Autodesk Fusion 360 part; units mm, degrees
(part 3 of 4)
extrude "Extrude14" cut sketch "left_side_misc" along normal up to surface (5.36 mm away) from surface at 107.32 contours A0 | A1 | A2 bodies 9
sketch "layer_0" plane through (0, 0, 0) normal (0, 1, 0) x (1, 0, 0)
  line L0 (-84.68, -41.5) -> (77.32, -41.5)
  line L1 (77.32, -41.5) -> (77.32, 105.5) construction
  line L2 (77.32, 105.5) -> (-84.68, 105.5)
  line L3 (-84.68, 105.5) -> (-84.68, -41.5)
  line L4 (38.25, 90) -> (38.25, -6)
  line L5 (38.25, 90) -> (77.32, 90)
  line L6 (38.25, -6) -> (77.32, -6)
  line L7 (77.32, 90) -> (77.32, 105.5)
  line L8 (77.32, -6) -> (77.32, -41.5)
  line L9 (72.32, -41.5) -> (72.32, -21.5) construction
  line L10 (72.32, -21.5) -> (77.32, -21.5) construction
  line L11 (-79.68, -41.5) -> (-79.68, -21.5) construction
  line L12 (-79.68, -21.5) -> (-84.68, -21.5) construction
  line L13 (-100, 100) -> (100, 100) construction
  line L14 (77.32, -6) -> (70.32, -6) construction
  line L15 (70.32, -6) -> (70.32, -13) construction
  line L16 (70.32, -13) -> (77.32, -13) construction
  line L17 (77.32, -13) -> (77.32, -6) construction
  line L18 (77.32, 90) -> (70.32, 90) construction
  line L19 (70.32, 90) -> (70.32, 97) construction
  line L20 (70.32, 97) -> (77.32, 97) construction
  line L21 (77.32, 97) -> (77.32, 90) construction
  line L22 (38.25, 90) -> (31.25, 90) construction
  line L23 (31.25, 90) -> (31.25, 97) construction
  line L24 (31.25, 97) -> (38.25, 97) construction
  line L25 (38.25, 97) -> (38.25, 90) construction
  line L26 (38.25, -6) -> (31.25, -6) construction
  line L27 (31.25, -6) -> (31.25, -13) construction
  line L28 (31.25, -13) -> (38.25, -13) construction
  line L29 (38.25, -13) -> (38.25, -6) construction
  line L30 (38.25, 97) -> (70.32, 97) construction
  line L31 (31.25, 90) -> (31.25, -6) construction
  line L32 (38.25, -13) -> (70.32, -13) construction
  line L33 (77.32, -9.5) -> (34.75, -9.5) construction
  line L34 (77.32, 93.5) -> (34.75, 93.5) construction
  line L35 (34.75, 93.5) -> (34.75, -9.5) construction
  line L36 (73.82, -9.5) -> (73.82, -13) construction
  line L37 (73.82, 97) -> (73.82, 93.5) construction
  line L38 (31.25, 97) -> (21.32, 97) construction
  line L39 (21.32, 97) -> (21.32, -13) construction
  line L40 (21.32, -13) -> (31.25, -13) construction
  line L41 (21.32, 42) -> (28.32, 42) construction
  line L42 (21.32, 5) -> (77.32, 5) construction
  line L43 (77.32, 90) -> (73.82, 90) construction
  line L44 (73.82, 90) -> (73.82, 86.5) construction
  line L45 (73.82, 86.5) -> (77.32, 86.5) construction
  line L46 (77.32, 86.5) -> (77.32, 90) construction
  line L47 (73.82, 86.5) -> (24.82, 86.5) construction
  line L48 (24.82, 86.5) -> (24.82, 28.5) construction
  line L49 (24.82, 28.5) -> (73.82, 28.5) construction
  line L50 (73.82, 28.5) -> (73.82, 86.5) construction
  line L51 (-84.68, 90) -> (-36.68, 90) construction
  line L52 (-36.68, 90) -> (-36.68, 21) construction
  line L53 (-36.68, 21) -> (-84.68, 21) construction
  line L54 (-84.68, 21) -> (-84.68, 90) construction
  line L55 (31.25, 90) -> (-84.68, 90) construction
  line L56 (-39.62, 23.94) -> (-81.74, 23.94) construction
  line L57 (-81.74, 23.94) -> (-81.74, 87.06) construction
  line L58 (-81.74, 87.06) -> (-39.62, 87.06) construction
  line L59 (-39.62, 87.06) -> (-39.62, 23.94) construction
  line L60 (-84.68, 90) -> (-81.74, 90) construction
  line L61 (-81.74, 90) -> (-81.74, 87.06) construction
  line L62 (-81.74, 87.06) -> (-84.68, 87.06) construction
  line L63 (-84.68, 87.06) -> (-84.68, 90) construction
  line L64 (-39.62, 23.94) -> (-36.68, 23.94) construction
  line L65 (-36.68, 23.94) -> (-36.68, 21) construction
  line L66 (-36.68, 21) -> (-39.62, 21) construction
  line L67 (-39.62, 21) -> (-39.62, 23.94) construction
  line L68 (-33.68, 17.618) -> (-1.422, 17.618) construction
  line L69 (-1.422, 17.618) -> (-1.422, -37.5) construction
  line L70 (-1.422, -37.5) -> (-33.68, -37.5) construction
  line L71 (-33.68, -37.5) -> (-33.68, 17.618) construction
  line L72 (-4.851, -34.071) -> (-30.251, -34.071) construction
  line L73 (-30.251, -34.071) -> (-30.251, 14.189) construction
  line L74 (-30.251, 14.189) -> (-4.851, 14.189) construction
  line L75 (-4.851, 14.189) -> (-4.851, -34.071) construction
  point P0 (-84.68, -41.5)
  point P1 (77.32, 105.5)
  point P2 (34.75, -6)
  point P3 (73.82, -9.5)
  point P4 (73.82, 93.5)
  point P5 (24.82, 42)
  dimension "d299" = 7
  dimension "d300" = 56
  dimension "d301" = 7
  dimension "d303" = 85
  dimension "d304" = 3.5
  dimension "d305" = 3.5
  dimension "d306" = 49
  dimension "d307" = 58
  dimension "d326" = 48
  dimension "d327" = 69
  dimension "d328" = 2.94
  dimension "d404" = 32.258
  dimension "d405" = 55.118
  dimension "d406" = 3.429
  dimension "d407" = 4
  dimension "d408" = 3
  constraint horizontal L0
  constraint vertical L1
  constraint horizontal L2
  constraint vertical L3
  constraint coincident P1 L1.end
  constraint coincident P0 L0.start
  constraint coincident L4.start L5.start
  constraint coincident L1 L5.end
  constraint perpendicular L1 L5
  constraint coincident L4.end L6.start
  constraint coincident L1 L6.end
  constraint perpendicular L1 L6
  constraint horizontal L14
  constraint vertical L15
  constraint horizontal L16
  constraint vertical L17
  constraint equal L15 L16
  constraint horizontal L18
  constraint vertical L19
  constraint horizontal L20
  constraint vertical L21
  constraint equal L19 L20
  constraint equal L15 L19
  constraint horizontal L22
  constraint vertical L23
  constraint horizontal L24
  constraint vertical L25
  constraint horizontal L26
  constraint vertical L27
  constraint horizontal L28
  constraint vertical L29
  constraint equal L15 L29
  constraint equal L26 L29
  constraint equal L22 L26
  constraint equal L22 L25
  constraint midpoint L17 L33.start
  constraint perpendicular L17 L33
  constraint midpoint L21 L34.start
  constraint perpendicular L25 L34
  constraint vertical L35
  constraint midpoint L26 P2
  constraint coincident L35 P2
  constraint coincident L33 P3
  constraint coincident P3 L36.start
  constraint midpoint L16 L36.end
  constraint vertical L36
  constraint midpoint L20 L37.start
  constraint coincident L34 P4
  constraint perpendicular L34 L37
  constraint coincident P4 L37.end
  constraint perpendicular L23 L38
  constraint perpendicular L22 L39
  constraint horizontal L40
  constraint midpoint L39 L41.start
  constraint perpendicular L39 L41
  constraint midpoint L41 P5
  constraint coincident L39 L42.start
  constraint coincident L1 L42.end
  constraint perpendicular L1 L42
  constraint horizontal L43
  constraint vertical L44
  constraint horizontal L45
  constraint vertical L46
  constraint horizontal L47
  constraint vertical L48
  constraint horizontal L49
  constraint vertical L50
  constraint coincident L3 L51.start
  constraint horizontal L51
  constraint vertical L52
  constraint horizontal L53
  constraint vertical L54
  constraint perpendicular L3 L55
  constraint coincident L51.start L54.end
  constraint horizontal L56
  constraint vertical L57
  constraint horizontal L58
  constraint vertical L59
  constraint horizontal L60
  constraint vertical L61
  constraint horizontal L62
  constraint vertical L63
  constraint horizontal L64
  constraint vertical L65
  constraint horizontal L66
  constraint vertical L67
  constraint equal L64 L67
  constraint equal L62 L64
  constraint equal L61 L62
  constraint horizontal L68
  constraint vertical L69
  constraint horizontal L70
  constraint vertical L71
  measures "d299" distance of L6.end L16.end
  measures "d300" distance of L20.end L38.end
  measures "d301" distance of L41.start L41.end
  measures "d303" distance of L5 L42
  measures "d304" distance of L5.end L43.end
  measures "d305" distance of L5.end L45.end
  measures "d306" distance of L44.end L47.end
  measures "d307" distance of L44.end L49.end
  measures "d326" distance of L51.start L51.end
  measures "d327" distance of L51.start L53.end
  measures "d328" distance of L56.start L66.end
  measures "d404" distance of L68.start L68.end
  measures "d405" distance of L68.end L69.end
  measures "d407" distance of L0 L70
  measures "d408" distance of L52 L71
sketch "layer_0_rpi_adapter" plane through (0, 0, 0) normal (0, 1, 0) x (1, 0, 0)
  line L0 (21.32, 97) -> (77.32, 97)
  line L1 (77.32, 97) -> (77.32, -13)
  line L2 (77.32, -13) -> (21.32, -13)
  line L3 (21.32, -13) -> (21.32, 97)
  line L4 (21.32, -13) -> (3.32, -13) construction
  line L5 (3.32, -13) -> (3.32, 97) construction
  line L6 (3.32, 97) -> (21.32, 97) construction
  point P0 (21.32, 97)
  point P1 (77.32, -13)
  dimension "d325" = 18
  constraint horizontal L0
  constraint vertical L1
  constraint horizontal L2
  constraint vertical L3
  constraint coincident P1 L1.end
  constraint coincident P0 L0.start
  constraint perpendicular L3 L4
  constraint perpendicular L4 L5
  constraint horizontal L6
  measures "d325" distance of L2.end L4.end
sketch "layer 0 planning" plane through (0, 0, 0) normal (0, 0, 1) x (1, 0, 0)
  line L0 (100, 42.675) -> (-100, 42.675)
  line L1 (100, 37.325) -> (-100, 37.325)
  line L2 (77.32, 42.675) -> (21.32, 42.675)
  line L3 (21.32, 42.675) -> (21.32, 47.675)
  line L4 (21.32, 47.675) -> (77.32, 47.675)
  line L5 (77.32, 47.675) -> (77.32, 42.675)
  line L6 (77.32, 47.675) -> (21.32, 47.675)
  line L7 (21.32, 47.675) -> (21.32, 53.025)
  line L8 (21.32, 53.025) -> (77.32, 53.025)
  line L9 (77.32, 53.025) -> (77.32, 47.675)
  line L10 (77.32, 53.025) -> (21.32, 53.025)
  line L11 (21.32, 53.025) -> (21.32, 58.025)
  line L12 (21.32, 58.025) -> (77.32, 58.025)
  line L13 (77.32, 58.025) -> (77.32, 53.025)
  line L14 (77.32, 58.025) -> (21.32, 58.025)
  line L15 (21.32, 58.025) -> (21.32, 76.025)
  line L16 (21.32, 76.025) -> (77.32, 76.025)
  line L17 (77.32, 76.025) -> (77.32, 58.025)
  point P0 (77.32, 0)
  point P1 (21.32, 0)
  dimension "d315" = 5
  dimension "d316" = 5.35
  dimension "d317" = 5
  dimension "d318" = 18
  constraint horizontal L2
  constraint vertical L3
  constraint horizontal L4
  constraint vertical L5
  constraint coincident L0 L2.start
  constraint vertical P1 L2.end
  constraint vertical P0 L2.start
  constraint horizontal L6
  constraint vertical L7
  constraint horizontal L8
  constraint vertical L9
  constraint vertical L3.end L7.end
  constraint horizontal L10
  constraint vertical L11
  constraint horizontal L12
  constraint vertical L13
  constraint vertical L7.end L11.end
  constraint horizontal L14
  constraint vertical L15
  constraint horizontal L16
  constraint vertical L17
  constraint vertical L11.end L15.end
  measures "d315" distance of L2.start L4.end
  measures "d316" distance of L4.end L8.end
  measures "d317" distance of L8.end L12.end
  measures "d318" distance of L12.end L16.end
extrude "Extrude21" add sketch "layer_0_rpi_adapter" along normal up to surface (5.35 mm away) from surface at 47.675 separate body makes body 12
extrude "Extrude22" add sketch "layer_0" along normal up to surface (5.35 mm away) from surface at 37.325 separate body makes body 13
hole "Hole6" at (73.82, 0, 9.5) at (34.75, 0, 9.5) at (24.82, 0, -42) at (34.75, 0, -93.5) at (73.82, 0, -93.5) at (-39.62, 0, -23.94) at (-39.62, 0, -87.06) at (-81.74, 0, -23.94) at (-81.74, 0, -87.06) at (-4.851, 0, 34.071) at (-4.851, 0, -14.189) at (-30.251, 0, -14.189) at (-30.251, 0, 34.071) direction (0, 1, 0) diameter 1.8 end up to surface (42.675 mm away) bodies 13
hole "Hole7" at (34.75, 0, -93.5) at (73.82, 0, -93.5) at (34.75, 0, 9.5) at (73.82, 0, 9.5) at (24.82, 0, -42) direction (0, 1, 0) diameter 2.8 end up to surface (53.025 mm away) bodies 4 12
hole "Hole8" at (24.82, 0, -86.5) at (24.82, 0, -28.5) at (73.82, 0, -28.5) at (73.82, 0, -86.5) direction (0, 1, 0) diameter 1.8 end up to surface (53.025 mm away) bodies 12
sketch "layer_0_laser" plane through (0, 42.675, 0) normal (0, 1, 0) x (-1, 0, 0)
  circle A0 centre (81.74, -23.94) radius 0.9
  circle A1 centre (39.62, -23.94) radius 0.9
  circle A2 centre (-34.75, -93.5) radius 0.9
  circle A3 centre (-34.75, 9.5) radius 0.9
  circle A4 centre (-73.82, 9.5) radius 0.9
  circle A5 centre (-24.82, -42) radius 0.9
  circle A6 centre (-73.82, -93.5) radius 0.9
  circle A7 centre (39.62, -87.06) radius 0.9
  circle A8 centre (81.74, -87.06) radius 0.9
  line L0 (-38.25, 6) -> (-38.25, -90)
  line L1 (-38.25, -90) -> (-77.32, -90)
  line L2 (-77.32, -90) -> (-77.32, -105.5)
  line L3 (-77.32, -105.5) -> (84.68, -105.5)
  line L4 (84.68, -105.5) -> (84.68, 41.5)
  line L5 (84.68, 41.5) -> (-77.32, 41.5)
  line L6 (-77.32, 41.5) -> (-77.32, 6)
  line L7 (-77.32, 6) -> (-38.25, 6)
  circle A9 centre (30.251, -14.189) radius 0.9
  circle A10 centre (4.851, 34.071) radius 0.9
  circle A11 centre (4.851, -14.189) radius 0.9
  circle A12 centre (30.251, 34.071) radius 0.9
sketch "layer_0_rpi_adapter_laser" plane through (0, 53.025, 0) normal (0, 1, 0) x (-1, 0, 0)
  circle A0 centre (-73.82, -28.5) radius 0.9
  circle A1 centre (-24.82, -86.5) radius 0.9
  circle A2 centre (-24.82, -28.5) radius 0.9
  circle A3 centre (-73.82, -86.5) radius 0.9
  circle A4 centre (-73.82, 9.5) radius 1.4
  circle A5 centre (-73.82, -93.5) radius 1.4
  circle A6 centre (-34.75, -93.5) radius 1.4
  circle A7 centre (-34.75, 9.5) radius 1.4
  circle A8 centre (-24.82, -42) radius 1.4
  line L0 (-21.32, -97) -> (-21.32, 13)
  line L1 (-21.32, 13) -> (-77.32, 13)
  line L2 (-77.32, 13) -> (-77.32, -97)
  line L3 (-77.32, -97) -> (-21.32, -97)
sketch "right_panel_laser" plane through (-112.68, 0, 0) normal (-1, 0, 0) x (0, 0, 1)
  circle A0 centre (32.8, 120) radius 2.5
  circle A1 centre (32.8, 199.925) radius 2.5
  circle A2 centre (32.8, 40.075) radius 2.5
  circle A3 centre (61, 170.495) radius 5
  circle A4 centre (37, 170.495) radius 5
  circle A5 centre (67, 180.8873) radius 5
  circle A6 centre (85, 191.28) radius 5
  circle A7 centre (85, 170.495) radius 5
  circle A8 centre (67, 139.3173) radius 5
  circle A9 centre (67, 118.5323) radius 5
  circle A10 centre (67, 97.7473) radius 5
  circle A11 centre (61, 108.14) radius 5
  circle A12 centre (55, 139.3173) radius 5
  circle A13 centre (49, 149.71) radius 5
  circle A14 centre (31, 160.1023) radius 5
  circle A15 centre (55, 160.1023) radius 5
  circle A16 centre (79, 160.1023) radius 5
  circle A17 centre (79, 139.3173) radius 5
  circle A18 centre (79, 118.5323) radius 5
  circle A19 centre (79, 97.7473) radius 5
  circle A20 centre (85, 87.355) radius 5
  circle A21 centre (85, 66.57) radius 5
  circle A22 centre (61, 87.355) radius 5
  circle A23 centre (67, 76.9623) radius 5
  circle A24 centre (61, 66.57) radius 5
  circle A25 centre (49, 66.57) radius 5
  circle A26 centre (67, 56.1773) radius 5
  circle A27 centre (85, 45.785) radius 5
  circle A28 centre (85, 25) radius 5
  circle A29 centre (61, 45.785) radius 5
  circle A30 centre (61, 25) radius 5
  circle A31 centre (37, 25) radius 5
  circle A32 centre (55, 35.3923) radius 5
  circle A33 centre (43, 56.1773) radius 5
  circle A34 centre (25, 66.57) radius 5
  circle A35 centre (49, 87.355) radius 5
  circle A36 centre (31, 76.9623) radius 5
  circle A37 centre (37, 87.355) radius 5
  circle A38 centre (19, 97.7473) radius 5
  circle A39 centre (43, 97.7473) radius 5
  circle A40 centre (55, 118.5323) radius 5
  circle A41 centre (43, 139.3173) radius 5
  circle A42 centre (19, 139.3173) radius 5
  circle A43 centre (19, 160.1023) radius 5
  circle A44 centre (19, 180.8873) radius 5
  circle A45 centre (43, 180.8873) radius 5
  circle A46 centre (61, 191.28) radius 5
  circle A47 centre (49, 191.28) radius 5
  circle A48 centre (31, 180.8873) radius 5
  circle A49 centre (25, 170.495) radius 5
  circle A50 centre (25, 149.71) radius 5
  circle A51 centre (31, 139.3173) radius 5
  circle A52 centre (49, 128.925) radius 5
  circle A53 centre (49, 108.14) radius 5
  circle A54 centre (31, 97.7473) radius 5
  circle A55 centre (25, 87.355) radius 5
  circle A56 centre (19, 76.9623) radius 5
  circle A57 centre (43, 76.9623) radius 5
  circle A58 centre (19, 56.1773) radius 5
  circle A59 centre (31, 56.1773) radius 5
  circle A60 centre (49, 45.785) radius 5
  circle A61 centre (49, 25) radius 5
  circle A62 centre (25, 25) radius 5
  circle A63 centre (67, 35.3923) radius 5
  circle A64 centre (73, 25) radius 5
  circle A65 centre (79, 35.3923) radius 5
  circle A66 centre (73, 45.785) radius 5
  circle A67 centre (55, 56.1773) radius 5
  circle A68 centre (37, 66.57) radius 5
  circle A69 centre (55, 76.9623) radius 5
  circle A70 centre (73, 66.57) radius 5
  circle A71 centre (79, 56.1773) radius 5
  circle A72 centre (79, 76.9623) radius 5
  circle A73 centre (73, 87.355) radius 5
  circle A74 centre (85, 108.14) radius 5
  circle A75 centre (85, 128.925) radius 5
  circle A76 centre (85, 149.71) radius 5
  circle A77 centre (67, 160.1023) radius 5
  circle A78 centre (43, 160.1023) radius 5
  circle A79 centre (37, 149.71) radius 5
  circle A80 centre (61, 149.71) radius 5
  circle A81 centre (61, 128.925) radius 5
  circle A82 centre (55, 97.7473) radius 5
  circle A83 centre (73, 108.14) radius 5
  circle A84 centre (73, 128.925) radius 5
  circle A85 centre (73, 149.71) radius 5
  circle A86 centre (79, 180.8873) radius 5
  circle A87 centre (73, 191.28) radius 5
  circle A88 centre (55, 180.8873) radius 5
  circle A89 centre (49, 170.495) radius 5
  circle A90 centre (73, 170.495) radius 5
  line L0 (105.5, 215.5) -> (-105.5, 215.5)
  line L1 (-105.5, 215.5) -> (-105.5, 4.5)
  line L2 (-105.5, 4.5) -> (105.5, 4.5)
  line L3 (105.5, 4.5) -> (105.5, 215.5)
sketch "left_panel_laser" plane through (112.68, 0, 0) normal (1, 0, 0) x (0, 0, -1)
  circle A0 centre (-64, 29.5) radius 11.6
  circle A1 centre (-73.6, 41.5) radius 1.1
  circle A2 centre (-54.4, 17.5) radius 1.1
  circle A3 centre (-34.3, 120) radius 2.5
  circle A4 centre (-34.3, 199.925) radius 2.5
  circle A5 centre (-34.3, 40.075) radius 2.5
  line L0 (-105.5, 215.5) -> (-105.5, 4.5)
  line L1 (-105.5, 4.5) -> (105.5, 4.5)
  line L2 (105.5, 4.5) -> (105.5, 215.5)
  line L3 (105.5, 215.5) -> (-105.5, 215.5)
  circle A6 centre (14.25, 188.25) radius 2.5
  line L4 (10, 135.4047) -> (10, 169.5953)
  arc A7 (32.9047, 192.5) -> (10, 169.5953) centre (50, 152.5) ccw
  line L5 (32.9047, 192.5) -> (67.0953, 192.5)
  arc A8 (90, 169.5953) -> (67.0953, 192.5) centre (50, 152.5) ccw
  line L6 (90, 169.5953) -> (90, 135.4047)
  arc A9 (67.0953, 112.5) -> (90, 135.4047) centre (50, 152.5) ccw
  line L7 (67.0953, 112.5) -> (32.9047, 112.5)
  arc A10 (10, 135.4047) -> (32.9047, 112.5) centre (50, 152.5) ccw
  circle A11 centre (85.75, 90.75) radius 2.5
  circle A12 centre (85.75, 188.25) radius 2.5
  circle A13 centre (14.25, 90.75) radius 2.5
  circle A14 centre (14.25, 116.75) radius 2.5
  circle A15 centre (85.75, 116.75) radius 2.5
  arc A16 (32.9047, 95) -> (10, 72.0953) centre (50, 55) ccw
  line L8 (32.9047, 95) -> (67.0953, 95)
  arc A17 (90, 72.0953) -> (67.0953, 95) centre (50, 55) ccw
  line L9 (90, 72.0953) -> (90, 37.9047)
  arc A18 (67.0953, 15) -> (90, 37.9047) centre (50, 55) ccw
  line L10 (67.0953, 15) -> (32.9047, 15)
  arc A19 (10, 37.9047) -> (32.9047, 15) centre (50, 55) ccw
  line L11 (10, 37.9047) -> (10, 72.0953)
  circle A20 centre (14.25, 19.25) radius 2.5
  circle A21 centre (85.75, 19.25) radius 2.5
sketch "left_panel_pcb_plan" plane through (107.32, 0, 0) normal (-1, 0, 0) x (0, 0, 1)
  circle A0 centre (64, 29.5) radius 11.6
  circle A1 centre (73.6, 41.5) radius 1.1
  circle A2 centre (54.4, 17.5) radius 1.1
  circle A3 centre (34.3, 120) radius 2.5
  circle A4 centre (34.3, 199.925) radius 2.5
  circle A5 centre (34.3, 40.075) radius 2.5
  circle A6 centre (-14.25, 188.25) radius 2.5
  arc A7 (-10, 169.5953) -> (-32.9047, 192.5) centre (-50, 152.5) ccw
  line L0 (-10, 169.5953) -> (-10, 135.4047)
  arc A8 (-32.9047, 112.5) -> (-10, 135.4047) centre (-50, 152.5) ccw
  line L1 (-32.9047, 112.5) -> (-67.0953, 112.5)
  arc A9 (-90, 135.4047) -> (-67.0953, 112.5) centre (-50, 152.5) ccw
  line L2 (-90, 135.4047) -> (-90, 169.5953)
  arc A10 (-67.0953, 192.5) -> (-90, 169.5953) centre (-50, 152.5) ccw
  line L3 (-67.0953, 192.5) -> (-32.9047, 192.5)
  circle A11 centre (-85.75, 90.75) radius 2.5
  circle A12 centre (-85.75, 188.25) radius 2.5
  circle A13 centre (-14.25, 90.75) radius 2.5
  circle A14 centre (-14.25, 116.75) radius 2.5
  circle A15 centre (-85.75, 116.75) radius 2.5
  line L4 (-67.0953, 95) -> (-32.9047, 95)
  arc A16 (-10, 72.0953) -> (-32.9047, 95) centre (-50, 55) ccw
  line L5 (-10, 72.0953) -> (-10, 37.9047)
  arc A17 (-32.9047, 15) -> (-10, 37.9047) centre (-50, 55) ccw
  line L6 (-32.9047, 15) -> (-67.0953, 15)
  arc A18 (-90, 37.9047) -> (-67.0953, 15) centre (-50, 55) ccw
  line L7 (-90, 37.9047) -> (-90, 72.0953)
  arc A19 (-67.0953, 95) -> (-90, 72.0953) centre (-50, 55) ccw
  circle A20 centre (-14.25, 19.25) radius 2.5
  circle A21 centre (-85.75, 19.25) radius 2.5
  line L8 (-105.5, 4.5) -> (105.5, 4.5)
  line L9 (105.5, 4.5) -> (105.5, 215.5)
  line L10 (105.5, 215.5) -> (-105.5, 215.5)
  line L11 (-105.5, 215.5) -> (-105.5, 4.5)
  line L12 (77, 45) -> (51, 45) construction
  line L13 (77, 14) -> (77, 45) construction
  line L14 (51, 45) -> (51, 14) construction
  line L15 (51, 14) -> (77, 14) construction
  line L16 (47.1, 49.075) -> (47.1, 31.075) construction
  line L17 (21.5, 49.075) -> (47.1, 49.075) construction
  line L18 (47.1, 127.5) -> (47.1, 112.5) construction
  line L19 (21.5, 127.5) -> (47.1, 127.5) construction
  line L20 (21.5, 208.925) -> (47.1, 208.925) construction
  line L21 (47.1, 208.925) -> (47.1, 190.925) construction
  line L22 (21.5, 208.925) -> (21.5, 190.925) construction
  line L23 (21.5, 31.075) -> (21.5, 49.075) construction
  line L24 (21.5, 112.5) -> (21.5, 127.5) construction
  line L25 (21.5, 31.075) -> (47.1, 31.075) construction
  line L26 (21.5, 112.5) -> (47.1, 112.5) construction
  line L27 (21.5, 190.925) -> (47.1, 190.925) construction
  line L28 (-10, 112.5) -> (-10, 192.5) construction
  line L29 (-10, 15) -> (-10, 95) construction
  line L30 (100, 210) -> (100, 10) construction
  line L31 (100, 10) -> (-100, 10) construction
  line L32 (-100, 210) -> (100, 210) construction
  line L33 (-97, 53.025) -> (13, 53.025) construction
  line L34 (-97, 53.025) -> (-97, 64.025) construction
  line L35 (-97, 64.025) -> (13, 64.025) construction
  line L36 (13, 64.025) -> (13, 53.025) construction
  line L37 (-7.5, 51.575) -> (97.5, 51.575) construction
  line L38 (97.5, 51.575) -> (97.5, 110) construction
  line L39 (97.5, 110) -> (-7.5, 110) construction
  line L40 (-7.5, 110) -> (-7.5, 51.575) construction
  line L41 (97.5, 188.425) -> (-7.5, 188.425) construction
  line L42 (-7.5, 188.425) -> (-7.5, 130) construction
  line L43 (-7.5, 130) -> (97.5, 130) construction
  line L44 (97.5, 130) -> (97.5, 188.425) construction
  line L45 (97.5, 110) -> (97.5, 130) construction
  line L46 (49.6, 110) -> (49.6, 130) construction
  line L47 (-7.5, 110) -> (-7.5, 130) construction
  line L48 (19, 110) -> (19, 130) construction
  line L49 (49.6, 188.425) -> (49.6, 207.5) construction
  line L50 (49.6, 207.5) -> (97.5, 207.5) construction
  line L51 (97.5, 207.5) -> (97.5, 188.425) construction
  line L52 (19, 188.425) -> (19, 207.5) construction
  line L53 (19, 207.5) -> (-7.5, 207.5) construction
  line L54 (-7.5, 207.5) -> (-7.5, 188.425) construction
  line L55 (19, 51.575) -> (19, 12.5) construction
  line L56 (19, 12.5) -> (-7.5, 12.5) construction
  line L57 (-7.5, 12.5) -> (-7.5, 51.575) construction
  line L58 (79.5, 51.575) -> (79.5, 12.5) construction
  line L59 (79.5, 12.5) -> (97.5, 12.5) construction
  line L60 (97.5, 12.5) -> (97.5, 51.575) construction
  line L61 (49.6, 110) -> (49.6, 51.575) construction
  line L62 (19, 110) -> (19, 51.575) construction
  line L63 (49.6, 130) -> (49.6, 188.425) construction
  line L64 (19, 188.425) -> (19, 130) construction
  dimension "d347" = 11
  dimension "d348" = 2.5
  dimension "d349" = 2.5
  dimension "d350" = 2.5
  dimension "d351" = 2.5
  dimension "d352" = 2.5
  dimension "d353" = 2.5
  dimension "d354" = 2.5
  dimension "d355" = 2.5
  dimension "d356" = 2.5
  dimension "d357" = 2.5
  dimension "d358" = 2.5
  dimension "d359" = 2.5
  dimension "d360" = 2.5
  dimension "d362" = 2.5
  dimension "d363" = 2.5
  dimension "d364" = 2.5
  constraint vertical L34
  constraint horizontal L35
  constraint vertical L36
  constraint coincident L33.end L36.end
  constraint coincident L33.start L34.start
  constraint horizontal L37
  constraint vertical L38
  constraint horizontal L39
  constraint vertical L40
  constraint horizontal L41
  constraint vertical L42
  constraint horizontal L43
  constraint vertical L44
  constraint coincident L39 L46.start
  constraint coincident L43 L46.end
  constraint perpendicular L43 L46
  constraint coincident L39 L48.start
  constraint coincident L43 L48.end
  constraint perpendicular L43 L48
  constraint vertical L49
  constraint horizontal L50
  constraint vertical L51
  constraint vertical L52
  constraint horizontal L53
  constraint vertical L54
  constraint vertical L55
  constraint horizontal L56
  constraint vertical L57
  constraint vertical L58
  constraint horizontal L59
  constraint vertical L60
  constraint collinear L56 L59
  constraint collinear L50 L53
  constraint coincident L37 L58.start
  constraint coincident L37 L55.start
  constraint coincident L41 L49.start
  constraint coincident L41 L52.start
  constraint coincident L37 L61.end
  constraint perpendicular L37 L61
  measures "d347" distance of L33.start L34.end
  measures "d348" distance of L17 L37
  measures "d349" distance of L29 L40
  measures "d350" distance of L26 L39
  measures "d351" distance of L30 L38
  measures "d352" distance of L30 L44
  measures "d353" distance of L28 L42
  measures "d354" distance of L19 L43
  measures "d355" distance of L27 L41
  measures "d356" distance of L18 L46
  measures "d357" distance of L24 L48
  measures "d358" distance of L21 L49
  measures "d359" distance of L32 L50
  measures "d360" distance of L22 L52
  measures "d362" distance of L23 L55
  measures "d363" distance of L13 L58
  measures "d364" distance of L31 L59
sketch "layer_1" plane through (0, 0, 0) normal (0, 1, 0) x (1, 0, 0)
  line L0 (-84.68, 105.5) -> (77.32, 105.5)
  line L1 (77.32, 105.5) -> (77.32, -41.5)
  line L2 (77.32, -41.5) -> (-84.68, -41.5)
  line L3 (-84.68, -41.5) -> (-84.68, 105.5)
  line L4 (21.32, 97) -> (21.32, -13) construction
  line L5 (38.25, -6) -> (77.32, -6) construction
  line L6 (38.25, -6) -> (21.32, -6) construction
  line L7 (21.32, -6) -> (18.32, -6)
  line L8 (18.32, -6) -> (18.32, 2)
  line L9 (18.32, 2) -> (21.32, 2)
  line L10 (21.32, 2) -> (21.32, -6)
  line L11 (24.32, 63.5) -> (-31.68, 63.5) construction
  line L12 (-31.68, 63.5) -> (-31.68, -21.5) construction
  line L13 (-31.68, -21.5) -> (24.32, -21.5) construction
  line L14 (24.32, -21.5) -> (24.32, 63.5) construction
  line L15 (-3.68, -41.5) -> (-3.68, -21.5) construction
  line L16 (-31.68, 63.5) -> (-28.74, 63.5) construction
  line L17 (-28.74, 63.5) -> (-28.74, 60.56) construction
  line L18 (-28.74, 60.56) -> (-31.68, 60.56) construction
  line L19 (-31.68, 60.56) -> (-31.68, 63.5) construction
  line L20 (24.32, 60.56) -> (21.38, 60.56) construction
  line L21 (21.38, 60.56) -> (21.38, 63.5) construction
  line L22 (-31.68, -18.56) -> (-28.74, -18.56) construction
  line L23 (-28.74, -18.56) -> (-28.74, -21.5) construction
  line L24 (21.38, -21.5) -> (21.38, -18.56) construction
  line L25 (21.38, -18.56) -> (24.32, -18.56) construction
  point P0 (-84.68, 105.5)
  point P1 (77.32, -41.5)
  dimension "d365" = 3
  dimension "d366" = 8
  dimension "d367" = 56
  dimension "d368" = 85
  dimension "d369" = 2.94
  dimension "d371" = 20
  constraint horizontal L0
  constraint vertical L1
  constraint horizontal L2
  constraint vertical L3
  constraint coincident P1 L1.end
  constraint coincident P0 L0.start
  constraint coincident L5.start L6.start
  constraint coincident L4 L6.end
  constraint perpendicular L4 L6
  constraint horizontal L7
  constraint vertical L8
  constraint horizontal L9
  constraint vertical L10
  constraint horizontal L11
  constraint vertical L12
  constraint horizontal L13
  constraint vertical L14
  constraint midpoint L2 L15.start
  constraint midpoint L13 L15.end
  constraint vertical L15
  constraint horizontal L16
  constraint vertical L17
  constraint horizontal L18
  constraint vertical L19
  constraint equal L17 L18
  constraint coincident L14 L20.start
  constraint perpendicular L14 L20
  constraint coincident L11 L21.end
  constraint perpendicular L11 L21
  constraint equal L20 L21
  constraint equal L17 L21
  constraint coincident L12 L22.start
  constraint perpendicular L12 L22
  constraint coincident L13 L23.end
  constraint perpendicular L13 L23
  constraint coincident L13 L24.start
  constraint perpendicular L13 L24
  constraint coincident L14 L25.end
  constraint perpendicular L14 L25
  constraint equal L22 L23
  constraint equal L24 L25
  constraint equal L23 L24
  constraint equal L18 L22
  measures "d365" distance of L6.end L7.end
  measures "d366" distance of L6.end L9.end
  measures "d367" distance of L11.start L11.end
  measures "d368" distance of L11.start L13.end
  measures "d369" distance of L11.end L16.end
  measures "d371" distance of L15.start L15.end
extrude "Extrude23" add sketch "layer_1" along normal up to surface (5.35 mm away) from surface at 77.325 separate body makes body 14
hole "Hole9" at (-28.74, 0, 18.56) at (-28.74, 0, -60.56) at (21.38, 0, -60.56) at (21.38, 0, 18.56) direction (0, 1, 0) diameter 1.8 end through all bodies 14
sketch "layer_1_laser" plane through (0, 82.675, 0) normal (0, 1, 0) x (-1, 0, 0)
  circle A0 centre (-21.38, -60.56) radius 0.9
  circle A1 centre (28.74, 18.56) radius 0.9
  circle A2 centre (28.74, -60.56) radius 0.9
  circle A3 centre (-21.38, 18.56) radius 0.9
  line L0 (-18.32, 6) -> (-18.32, -2)
  line L1 (-18.32, -2) -> (-21.32, -2)
  line L2 (-21.32, -2) -> (-21.32, 6)
  line L3 (-21.32, 6) -> (-18.32, 6)
  line L4 (84.68, -105.5) -> (84.68, 41.5)
  line L5 (84.68, 41.5) -> (-77.32, 41.5)
  line L6 (-77.32, 41.5) -> (-77.32, -105.5)
  line L7 (-77.32, -105.5) -> (84.68, -105.5)
sketch "right_panel_pcb_plan" plane through (-107.32, 0, 0) normal (1, 0, 0) x (0, 0, -1)
  circle A0 centre (-32.8, 199.925) radius 2.5 construction
  circle A1 centre (-32.8, 40.075) radius 2.5 construction
  circle A2 centre (-61, 170.495) radius 5 construction
  circle A3 centre (-37, 170.495) radius 5 construction
  circle A4 centre (-67, 180.8873) radius 5 construction
  circle A5 centre (-85, 191.28) radius 5 construction
  circle A6 centre (-85, 170.495) radius 5 construction
  circle A7 centre (-55, 160.1023) radius 5 construction
  circle A8 centre (-79, 160.1023) radius 5 construction
  circle A9 centre (-61, 25) radius 5 construction
  circle A10 centre (-37, 25) radius 5 construction
  circle A11 centre (-55, 35.3923) radius 5 construction
  circle A12 centre (-43, 56.1773) radius 5 construction
  circle A13 centre (-25, 66.57) radius 5 construction
  circle A14 centre (-19, 97.7473) radius 5
  circle A15 centre (-43, 97.7473) radius 5
  circle A16 centre (-43, 139.3173) radius 5
  circle A17 centre (-19, 139.3173) radius 5
  circle A18 centre (-19, 180.8873) radius 5 construction
  circle A19 centre (-43, 180.8873) radius 5 construction
  circle A20 centre (-61, 191.28) radius 5 construction
  circle A21 centre (-49, 191.28) radius 5 construction
  circle A22 centre (-31, 180.8873) radius 5 construction
  circle A23 centre (-25, 170.495) radius 5 construction
  circle A24 centre (-49, 128.925) radius 5
  circle A25 centre (-49, 108.14) radius 5 construction
  circle A26 centre (-19, 76.9623) radius 5 construction
  circle A27 centre (-19, 56.1773) radius 5 construction
  circle A28 centre (-31, 56.1773) radius 5 construction
  circle A29 centre (-49, 45.785) radius 5 construction
  circle A30 centre (-49, 25) radius 5 construction
  circle A31 centre (-25, 25) radius 5 construction
  circle A32 centre (-67, 35.3923) radius 5 construction
  circle A33 centre (-73, 25) radius 5 construction
  circle A34 centre (-85, 149.71) radius 5 construction
  circle A35 centre (-67, 160.1023) radius 5 construction
  circle A36 centre (-43, 160.1023) radius 5 construction
  circle A37 centre (-61, 149.71) radius 5 construction
  circle A38 centre (-73, 149.71) radius 5 construction
  circle A39 centre (-79, 180.8873) radius 5 construction
  circle A40 centre (-73, 191.28) radius 5 construction
  circle A41 centre (-55, 180.8873) radius 5 construction
  circle A42 centre (-49, 170.495) radius 5 construction
  circle A43 centre (-73, 170.495) radius 5 construction
  line L0 (105.5, 4.5) -> (105.5, 215.5)
  line L1 (105.5, 215.5) -> (-105.5, 215.5)
  line L2 (-105.5, 215.5) -> (-105.5, 4.5)
  line L3 (-105.5, 4.5) -> (105.5, 4.5) construction
  circle A44 centre (-19, 180.8873) radius 5 construction
  circle A45 centre (-19, 139.3173) radius 5 construction
  circle A46 centre (-19, 97.7473) radius 5 construction
  circle A47 centre (-43, 97.7473) radius 5 construction
  circle A48 centre (-49, 108.14) radius 5 construction
  circle A49 centre (-49, 128.925) radius 5 construction
  circle A50 centre (-43, 139.3173) radius 5 construction
  circle A51 centre (-19, 56.1773) radius 5 construction
  circle A52 centre (-25, 25) radius 5 construction
  circle A53 centre (-49, 25) radius 5 construction
  circle A54 centre (-49, 45.785) radius 5 construction
  circle A55 centre (-43, 56.1773) radius 5 construction
  circle A56 centre (-43, 180.8873) radius 5 construction
  circle A57 centre (-49, 191.28) radius 5 construction
  line L4 (-21.5, 112.5) -> (-21.5, 127.5) construction
  line L5 (-21.5, 127.5) -> (-44.1, 127.5) construction
  line L6 (-21.5, 208.925) -> (-21.5, 190.925) construction
  line L7 (-21.5, 31.075) -> (-21.5, 49.075) construction
  line L8 (-21.5, 49.075) -> (-44.1, 49.075) construction
  line L9 (-21.5, 208.925) -> (-44.1, 208.925) construction
  line L10 (-21.5, 31.075) -> (-44.1, 31.075) construction
  line L11 (-21.5, 112.5) -> (-44.1, 112.5) construction
  line L12 (-21.5, 190.925) -> (-44.1, 190.925) construction
  line L13 (100, 210) -> (-100, 210) construction
  line L14 (100, 10) -> (100, 210) construction
  line L15 (-100, 10) -> (100, 10) construction
  line L16 (100, 210) -> (97.5, 210) construction
  line L17 (97.5, 210) -> (97.5, 207.5) construction
  line L18 (97.5, 207.5) -> (100, 207.5) construction
  line L19 (100, 207.5) -> (100, 210) construction
  line L20 (100, 10) -> (97.5, 10) construction
  line L21 (97.5, 10) -> (97.5, 12.5) construction
  line L22 (97.5, 12.5) -> (100, 12.5) construction
  line L23 (100, 12.5) -> (100, 10) construction
  line L24 (-14, 210) -> (-14, 10) construction
  line L25 (97.5, 12.5) -> (-11.5, 12.5) construction
  line L26 (-11.5, 12.5) -> (-11.5, 207.5) construction
  line L27 (-11.5, 207.5) -> (97.5, 207.5) construction
  line L28 (97.5, 207.5) -> (97.5, 12.5) construction
  line L29 (71.5, 187.5) -> (14.5, 187.5) construction
  line L30 (14.5, 187.5) -> (14.5, 158) construction
  line L31 (14.5, 158) -> (71.5, 158) construction
  line L32 (71.5, 158) -> (71.5, 187.5) construction
  line L33 (43, 207.5) -> (43, 187.5) construction
  line L34 (7.25, 192.3) -> (78.25, 192.3) construction
  line L35 (78.25, 192.3) -> (78.25, 149.3) construction
  line L36 (78.25, 149.3) -> (7.25, 149.3) construction
  line L37 (7.25, 149.3) -> (7.25, 192.3) construction
  line L38 (11.95, 189.5) -> (74.05, 189.5) construction
  line L39 (74.05, 189.5) -> (74.05, 150.7) construction
  line L40 (74.05, 150.7) -> (11.95, 150.7) construction
  line L41 (11.95, 150.7) -> (11.95, 189.5) construction
  line L42 (76.35, 151.2) -> (9.15, 151.2) construction
  line L43 (9.15, 151.2) -> (9.15, 190.4) construction
  line L44 (9.15, 190.4) -> (76.35, 190.4) construction
  line L45 (76.35, 190.4) -> (76.35, 151.2) construction
  line L46 (14, 157.5) -> (72, 157.5)
  line L47 (72, 157.5) -> (72, 188)
  line L48 (72, 188) -> (14, 188)
  line L49 (14, 188) -> (14, 157.5)
  circle A58 centre (9.15, 190.4) radius 0.9
  circle A59 centre (76.35, 190.4) radius 0.9
  circle A60 centre (76.35, 151.2) radius 0.9
  circle A61 centre (9.15, 151.2) radius 0.9
  line L50 (93, 176.5) -> (-7, 176.5) construction
  line L51 (-7, 176.5) -> (-7, 26.5) construction
  line L52 (-7, 26.5) -> (93, 26.5) construction
  line L53 (93, 26.5) -> (93, 176.5) construction
  line L54 (43, 187.5) -> (43, 176.5) construction
  line L55 (80.25, 176.5) -> (80.25, 147.3) construction
  line L56 (80.25, 147.3) -> (-7, 147.3) construction
  line L57 (80.25, 147.3) -> (78.25, 147.3) construction
  line L58 (78.25, 147.3) -> (78.25, 149.3) construction
  line L59 (78.25, 149.3) -> (80.25, 149.3) construction
  line L60 (80.25, 149.3) -> (80.25, 147.3) construction
  line L61 (87.25, 168.375) -> (81.25, 168.375) construction
  line L62 (81.25, 168.375) -> (81.25, 162.375) construction
  line L63 (81.25, 162.375) -> (87.25, 162.375) construction
  line L64 (87.25, 162.375) -> (87.25, 168.375) construction
  line L65 (71.5, 172.75) -> (71.5, 158) construction
  line L66 (71.5, 165.375) -> (81.25, 165.375) construction
  line L67 (84.25, 168.375) -> (84.25, 162.375) construction
  line L68 (71.5, 158) -> (43, 158) construction
  line L69 (57.25, 158) -> (57.25, 147.3) construction
  line L70 (71.5, 158) -> (71.5, 147.3) construction
  line L71 (43, 158) -> (43, 147.3) construction
  line L72 (43, 158) -> (14.5, 158) construction
  line L73 (14.5, 158) -> (14.5, 147.3) construction
  line L74 (28.75, 158) -> (28.75, 147.3) construction
  line L75 (67.375, 146.3) -> (61.375, 146.3) construction
  line L76 (61.375, 146.3) -> (61.375, 140.3) construction
  line L77 (61.375, 140.3) -> (67.375, 140.3) construction
  line L78 (67.375, 140.3) -> (67.375, 146.3) construction
  line L79 (53.125, 146.3) -> (47.125, 146.3) construction
  line L80 (47.125, 146.3) -> (47.125, 140.3) construction
  line L81 (47.125, 140.3) -> (53.125, 140.3) construction
  line L82 (53.125, 140.3) -> (53.125, 146.3) construction
  line L83 (38.875, 146.3) -> (32.875, 146.3) construction
  line L84 (32.875, 146.3) -> (32.875, 140.3) construction
  line L85 (32.875, 140.3) -> (38.875, 140.3) construction
  line L86 (38.875, 140.3) -> (38.875, 146.3) construction
  line L87 (24.625, 146.3) -> (18.625, 146.3) construction
  line L88 (18.625, 146.3) -> (18.625, 140.3) construction
  line L89 (18.625, 140.3) -> (24.625, 140.3) construction
  line L90 (24.625, 140.3) -> (24.625, 146.3) construction
  line L91 (71.5, 147.3) -> (57.25, 147.3) construction
  line L92 (57.25, 147.3) -> (43, 147.3) construction
  line L93 (43, 147.3) -> (28.75, 147.3) construction
  line L94 (14.5, 147.3) -> (28.75, 147.3) construction
  line L95 (21.625, 147.3) -> (21.625, 146.3) construction
  line L96 (35.875, 147.3) -> (35.875, 146.3) construction
  line L97 (50.125, 147.3) -> (50.125, 146.3) construction
  line L98 (64.375, 147.3) -> (64.375, 146.3) construction
  line L99 (67.375, 143.3) -> (61.375, 143.3) construction
  line L100 (53.125, 143.3) -> (47.125, 143.3) construction
  line L101 (38.875, 143.3) -> (32.875, 143.3) construction
  line L102 (24.625, 143.3) -> (18.625, 143.3) construction
  line L103 (93, 137.3) -> (-7, 137.3) construction
  line L104 (93, 125.3) -> (-7, 125.3) construction
  line L105 (93, 113.3) -> (-7, 113.3) construction
  line L106 (93, 101.3) -> (-7, 101.3) construction
  line L107 (93, 89.3) -> (-7, 89.3) construction
  line L108 (93, 77.3) -> (-7, 77.3) construction
  line L109 (93, 65.3) -> (-7, 65.3) construction
  line L110 (93, 53.3) -> (-7, 53.3) construction
  line L111 (93, 41.3) -> (-7, 41.3) construction
  line L112 (93, 29.3) -> (-7, 29.3) construction
  line L113 (85, 137.3) -> (85, 29.3) construction
  line L114 (93, 29.3) -> (85, 29.3) construction
  line L115 (1, 29.3) -> (1, 137.3) construction
  line L116 (1, 29.3) -> (-7, 29.3) construction
  line L117 (85, 137.3) -> (68.2, 137.3) construction
  line L118 (68.2, 137.3) -> (51.4, 137.3) construction
  line L119 (51.4, 137.3) -> (34.6, 137.3) construction
  line L120 (34.6, 137.3) -> (17.8, 137.3) construction
  line L121 (17.8, 137.3) -> (1, 137.3) construction
  line L122 (68.2, 137.3) -> (68.2, 29.3) construction
  line L123 (51.4, 137.3) -> (51.4, 29.3) construction
  line L124 (34.6, 137.3) -> (34.6, 29.3) construction
  line L125 (17.8, 137.3) -> (17.8, 17.7936) construction
  line L126 (56.8, 35.3) -> (62.8, 35.3) construction
  line L127 (62.8, 35.3) -> (62.8, 41.3) construction
  line L128 (62.8, 41.3) -> (56.8, 41.3) construction
  line L129 (56.8, 41.3) -> (56.8, 35.3) construction
  line L130 (23.2, 35.3) -> (29.2, 35.3) construction
  line L131 (29.2, 35.3) -> (29.2, 41.3) construction
  line L132 (29.2, 41.3) -> (23.2, 41.3) construction
  line L133 (23.2, 41.3) -> (23.2, 35.3) construction
  line L134 (68.2, 41.3) -> (51.4, 41.3) construction
  line L135 (34.6, 41.3) -> (17.8, 41.3) construction
  line L136 (62.8, 38.3) -> (56.8, 38.3) construction
  line L137 (29.2, 38.3) -> (23.2, 38.3) construction
  line L138 (59.8, 38.3) -> (59.8, 45.8) construction
  line L139 (26.2, 38.3) -> (26.2, 45.8) construction
  line L140 (34.6, 53.3) -> (51.4, 65.3) construction
  line L141 (34.6, 89.3) -> (51.4, 101.3) construction
  line L142 (51.4, 137.3) -> (34.6, 125.3) construction
  line L143 (85, 77.3) -> (68.2, 77.3) construction
  line L144 (68.2, 77.3) -> (51.4, 77.3) construction
  line L145 (51.4, 77.3) -> (34.6, 77.3) construction
  line L146 (34.6, 77.3) -> (17.8, 77.3) construction
  line L147 (17.8, 77.3) -> (1, 77.3) construction
  line L148 (85, 113.3) -> (68.2, 113.3) construction
  line L149 (68.2, 113.3) -> (51.4, 113.3) construction
  line L150 (51.4, 113.3) -> (34.6, 113.3) construction
  line L151 (34.6, 113.3) -> (17.8, 113.3) construction
  line L152 (17.8, 113.3) -> (1, 113.3) construction
  line L153 (62.8, 77.3) -> (56.8, 77.3) construction
  line L154 (56.8, 77.3) -> (56.8, 71.3) construction
  line L155 (56.8, 71.3) -> (62.8, 71.3) construction
  line L156 (62.8, 71.3) -> (62.8, 77.3) construction
  line L157 (29.2, 77.3) -> (23.2, 77.3) construction
  line L158 (23.2, 77.3) -> (23.2, 71.3) construction
  line L159 (23.2, 71.3) -> (29.2, 71.3) construction
  line L160 (29.2, 71.3) -> (29.2, 77.3) construction
  line L161 (62.8, 113.3) -> (56.8, 113.3) construction
  line L162 (56.8, 113.3) -> (56.8, 107.3) construction
  line L163 (56.8, 107.3) -> (62.8, 107.3) construction
  line L164 (62.8, 107.3) -> (62.8, 113.3) construction
  line L165 (29.2, 113.3) -> (23.2, 113.3) construction
  line L166 (23.2, 113.3) -> (23.2, 107.3) construction
  line L167 (23.2, 107.3) -> (29.2, 107.3) construction
  line L168 (29.2, 107.3) -> (29.2, 113.3) construction
  line L169 (62.8, 110.3) -> (56.8, 110.3) construction
  line L170 (29.2, 110.3) -> (23.2, 110.3) construction
  line L171 (29.2, 74.3) -> (23.2, 74.3) construction
  line L172 (62.8, 74.3) -> (56.8, 74.3) construction
  line L173 (59.8, 74.3) -> (59.8, 81.8) construction
  line L174 (26.2, 74.3) -> (26.2, 81.8) construction
  line L175 (59.8, 110.3) -> (59.8, 117.8) construction
  line L176 (26.2, 110.3) -> (26.2, 117.8) construction
  line L177 (79.6, 80.3) -> (73.6, 80.3) construction
  line L178 (73.6, 80.3) -> (73.6, 74.3) construction
  line L179 (73.6, 74.3) -> (79.6, 74.3) construction
  line L180 (79.6, 74.3) -> (79.6, 80.3) construction
  line L181 (46, 80.3) -> (40, 80.3) construction
  line L182 (40, 80.3) -> (40, 74.3) construction
  line L183 (40, 74.3) -> (46, 74.3) construction
  line L184 (46, 74.3) -> (46, 80.3) construction
  line L185 (12.4, 80.3) -> (6.4, 80.3) construction
  line L186 (6.4, 80.3) -> (6.4, 74.3) construction
  line L187 (6.4, 74.3) -> (12.4, 74.3) construction
  line L188 (12.4, 74.3) -> (12.4, 80.3) construction
  line L189 (80.3725, 116.2003) -> (72.8275, 116.2003) construction
  line L190 (72.8275, 116.2003) -> (72.8275, 110.3997) construction
  line L191 (72.8275, 110.3997) -> (80.3725, 110.3997) construction
  line L192 (80.3725, 110.3997) -> (80.3725, 116.2003) construction
  line L193 (47.1696, 117.2711) -> (38.8304, 117.2711) construction
  line L194 (38.8304, 117.2711) -> (38.8304, 109.3289) construction
  line L195 (38.8304, 109.3289) -> (47.1696, 109.3289) construction
  line L196 (47.1696, 109.3289) -> (47.1696, 117.2711) construction
  line L197 (12.5769, 117.2711) -> (6.2231, 117.2711) construction
  line L198 (6.2231, 117.2711) -> (6.2231, 109.3289) construction
  line L199 (6.2231, 109.3289) -> (12.5769, 109.3289) construction
  line L200 (12.5769, 109.3289) -> (12.5769, 117.2711) construction
  line L201 (79.6, 80.3) -> (73.6, 74.3) construction
  line L202 (46, 80.3) -> (40, 74.3) construction
  line L203 (12.4, 80.3) -> (6.4, 74.3) construction
  line L204 (12.5769, 117.2711) -> (6.2231, 109.3289) construction
  line L205 (47.1696, 117.2711) -> (38.8304, 109.3289) construction
  line L206 (80.3725, 116.2003) -> (72.8275, 110.3997) construction
  point P0 (-49, 108.14)
  point P1 (76.75, 163.18)
  point P2 (76.75, 165.72)
  point P3 (76.75, 168.26)
  point P4 (76.75, 170.8)
  point P5 (76.75, 173.34)
  point P6 (76.75, 175.88)
  point P7 (76.75, 178.42)
  point P8 (71.5, 172.75)
  point P9 (71.5, 165.375)
  point P10 (84.25, 165.375)
  point P11 (64.375, 143.3)
  point P12 (50.125, 143.3)
  point P13 (35.875, 143.3)
  point P14 (21.625, 143.3)
  point P15 (59.8, 41.3)
  point P16 (26.2, 41.3)
  dimension "d377" = 2.5
  dimension "d379" = 2.5
  dimension "d380" = 20
  dimension "d381" = 57
  dimension "d382" = 29.5
  dimension "d385" = 71
  dimension "d386" = 43
  dimension "d387" = 2
  dimension "d388" = 2.8
  dimension "d389" = 2.55
  dimension "d390" = 62.1
  dimension "d391" = 38.8
  dimension "d392" = 1.9
  dimension "d393" = 13.88
  dimension "d397" = 0
  dimension "d398" = 2.54
  dimension "d399" = 0.5
  dimension "d400" = 1.8
  dimension "d402" = 4.7
  dimension "d403" = 1.5
  dimension "d409" = 100
  dimension "d410" = 150
  dimension "d411" = 11
  dimension "d412" = 2
  dimension "d413" = 6
  dimension "d414" = 1
  dimension "d415" = 1
  dimension "d418" = 0
  dimension "d419" = -12
  dimension "d420" = 8
  dimension "d421" = 10
  dimension "d422" = 7.5
  constraint horizontal L16
  constraint vertical L17
  constraint horizontal L18
  constraint vertical L19
  constraint coincident L13.start L14.end
  constraint horizontal L20
  constraint vertical L21
  constraint horizontal L22
  constraint vertical L23
  constraint coincident L14.start L15.end
  constraint equal L17 L18
  constraint equal L18 L22
  constraint equal L21 L22
  constraint coincident L13 L24.start
  constraint coincident L15 L24.end
  constraint perpendicular L15 L24
  constraint tangent A17 L24
  constraint horizontal L25
  constraint vertical L26
  constraint horizontal L27
  constraint vertical L28
  constraint coincident L17.end L18.start
  constraint horizontal L29
  constraint vertical L30
  constraint horizontal L31
  constraint vertical L32
  constraint midpoint L27 L33.start
  constraint midpoint L29 L33.end
  constraint vertical L33
  constraint horizontal L34
  constraint vertical L35
  constraint horizontal L36
  constraint vertical L37
  constraint horizontal L38
  constraint vertical L39
  constraint horizontal L40
  constraint vertical L41
  constraint coincident L43.end L44.start
  constraint coincident L44.end L45.start
  constraint coincident L42.start L45.end
  constraint coincident L42.end L43.start
  constraint equal A58 A61
  constraint equal A60 A61
  constraint equal A59 A60
  constraint horizontal L50
  constraint vertical L51
  constraint horizontal L52
  constraint vertical L53
  constraint midpoint L50 L54.end
  constraint vertical L54
  constraint coincident L50 L55.start
  constraint perpendicular L50 L55
  constraint coincident L51 L56.end
  constraint perpendicular L51 L56
  constraint horizontal L57
  constraint vertical L58
  constraint horizontal L59
  constraint vertical L60
  constraint equal L58 L59
  constraint horizontal L61
  constraint vertical L62
  constraint horizontal L63
  constraint vertical L64
  constraint equal L61 L64
  constraint midpoint L32 P8
  constraint coincident P8 L65.start
  constraint midpoint L65 P9
  constraint coincident P9 L66.start
  constraint midpoint L62 L66.end
  constraint horizontal L66
  constraint midpoint L61 L67.start
  constraint midpoint L63 L67.end
  constraint midpoint L67 P10
  constraint midpoint L31 L68.end
  constraint midpoint L68 L69.start
  constraint coincident L56 L69.end
  constraint perpendicular L56 L69
  constraint coincident L56 L70.end
  constraint perpendicular L56 L70
  constraint coincident L56 L71.end
  constraint perpendicular L56 L71
  constraint coincident L56 L73.end
  constraint perpendicular L56 L73
  constraint midpoint L72 L74.start
  constraint coincident L56 L74.end
  constraint perpendicular L56 L74
  constraint horizontal L75
  constraint vertical L76
  constraint horizontal L77
  constraint vertical L78
  constraint horizontal L79
  constraint vertical L80
  constraint horizontal L81
  constraint vertical L82
  constraint horizontal L83
  constraint vertical L84
  constraint horizontal L85
  constraint vertical L86
  constraint horizontal L87
  constraint vertical L88
  constraint horizontal L89
  constraint vertical L90
  constraint equal L63 L75
  constraint equal L75 L78
  constraint equal L76 L79
  constraint equal L79 L82
  constraint equal L79 L83
  constraint equal L79 L86
  constraint equal L83 L87
  constraint equal L87 L90
  constraint midpoint L94 L95.start